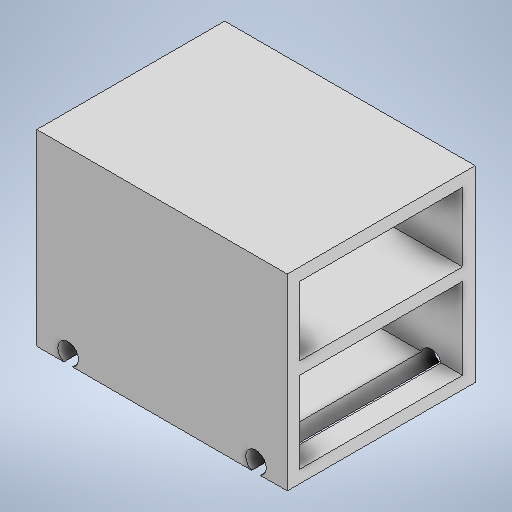
# Autodesk Inventor part: body
Saved by Autodesk Inventor 2025.3 (Build 293356030, 356C)
## iProperties
Created: 2026-06-23
Part Number: body
Material: Generic
Document SubType Name: Modeling
Designer: user
Density: 1 g/cm^3
Appearance: Default
Author: user
Autodesk Inventor part; units mm, degrees
ref_plane "YZ Plane" through (0, 0, 0) normal (1, 0, 0) x (0, 1, 0)
ref_plane "XZ Plane" through (0, 0, 0) normal (0, 1, 0) x (-1, 0, 0)
sketch "Sketch1" plane through (0, 0, 0) normal (0, 1, 0) x (-1, 0, 0)
  line L0 (0, 0) -> (-400, 0)
  line L1 (-400, 0) -> (-400, -300)
  line L2 (-400, -300) -> (0, -300)
  line L3 (0, -300) -> (0, 0)
  dimension "d0" = 400
  dimension "d1" = 300
  constraints: 8 end point, 2 parallel, 1 horizontal, 1 perpendicular
  measures "d0" distance of L2.end L1.end
  measures "d1" distance of L0.end L1.end
extrude "Extrusion1" add sketch "Sketch1" along normal blind 300
shell "Shell2" thickness 20 removed faces 2 at (0, 100, -200) at (400, 100, -100)
sketch "Sketch2" plane through (0, 0, 0) normal (0, 0, 1) x (1, 0, 0)
  circle A0 centre (50, 15) radius 16.5
  circle A1 centre (350, 15) radius 16.5
  line L0 (0, 0) -> (400, 0) projected
  dimension "d13" = 33
  dimension "d14" = 33
  dimension "d19" = 15
  dimension "d20" = 15
  constraints: 2 centre point
  measures "d13" diameter of A0
  measures "d14" diameter of A1
  measures "d19" distance from line of L0 A0.centre
  measures "d20" distance from line of L0 A1.centre
extrude "Extrusion2" cut sketch "Sketch2" against normal through all
ref_plane "Work Plane1" through (0, 160, 0) normal (0, 1, 0) x (1, 0, 0)
sketch "Sketch3" plane through (0, 160, 0) normal (0, 1, 0) x (1, 0, 0)
  line L0 (400, 300) -> (0, 300) projected
  line L1 (0, 300) -> (400, 300)
  line L2 (400, 300) -> (400, 0)
  line L3 (400, 0) -> (0, 0)
  line L4 (0, 0) -> (0, 300)
  constraints: 8 end point, 2 parallel, 1 horizontal, 1 perpendicular
extrude "Extrusion3" add sketch "Sketch3" along normal mid plane 20
body "Solid1"
